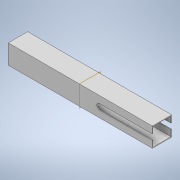
# Autodesk Inventor part: CatapultArmExtensionForRear
Saved by Autodesk Inventor 2022.2 (Build 262287000, 287)
## iProperties
Created: 2022-01-16
Part Number: CatapultArmExtensionForRear
Material: Generic
Document SubType Name: Modeling
Designer: robst
Density: 1 g/cm^3
Appearance: Default
Author: robst
Autodesk Inventor part; units mm, degrees
ref_plane "XZ Plane" through (0, 0, 0) normal (0, 1, 0) x (-1, 0, 0)
ref_plane "XY Plane" through (0, 0, 0) normal (0, 0, 1) x (1, 0, 0)
sketch "Sketch1" plane through (0, 0, 0) normal (0, 0, 1) x (1, 0, 0)
  line L0 (-330.2, -44.45) -> (330.2, -44.45)
  line L1 (330.2, 44.45) -> (-330.2, 44.45)
  line L2 (-330.2, 44.45) -> (-330.2, -44.45)
  line L3 (-330.2, -44.45) -> (330.2, 44.45) construction
  line L4 (330.2, -44.45) -> (-330.2, 44.45) construction
  line L5 (88.9, 0) -> (571.5, 0) construction
  line L6 (88.9, -12.7) -> (330.2, -12.7)
  line L7 (330.2, 12.7) -> (88.9, 12.7)
  arc A0 (88.9, 12.7) -> (88.9, -12.7) centre (88.9, 0) ccw
  line L8 (330.2, -44.45) -> (330.2, -12.7)
  line L9 (330.2, 12.7) -> (330.2, 44.45)
  point P0 (0, 0)
  point P1 (330.2, 0)
  point P2 (76.2, 0)
  dimension "d0" = 88.9
  dimension "d1" = 660.4
  dimension "d5" = 406.4
  dimension "d7" = 25.4
  constraints: 22 end point, 4 parallel, 4 perpendicular, 3 midpoint, 3 point on circle, 2 tangent, 1 centre point, 1 horizontal
  measures "d0" distance of L1.end L0.start
  measures "d1" distance of L1.start L1.end
  measures "d5" distance from line of point (76.2, 0) L2
  measures "d7" distance between parallel lines of L6 L7
extrude "Extrusion2" add sketch "Sketch1" along normal mid plane 88.9
sketch "Sketch2" plane through (0, 0, 0) normal (1, 0, 0) x (0, 1, 0)
  line L0 (-41.275, 41.275) -> (-41.275, -41.275)
  line L1 (-41.275, -41.275) -> (41.275, -41.275)
  line L2 (41.275, -41.275) -> (41.275, 41.275)
  line L3 (41.275, 41.275) -> (-41.275, 41.275)
  line L4 (-41.275, 41.275) -> (41.275, -41.275) construction
  line L5 (-41.275, -41.275) -> (41.275, 41.275) construction
  line L6 (44.45, -44.45) -> (44.45, 44.45) projected
  line L7 (44.45, 44.45) -> (-44.45, 44.45) projected
  point P0 (0, 0)
  dimension "d10" = 3.175
  dimension "d11" = 3.175
  constraints: 12 end point, 2 midpoint, 2 parallel, 1 perpendicular, 1 vertical
  measures "d10" distance between parallel lines of L2 L6
  measures "d11" distance between parallel lines of L3 L7
extrude "Extrusion3" cut sketch "Sketch2" along normal through all both and the other way through all
body "Solid2"
